Autodesk Fusion 360 part; units mm, degrees
(part 6 of 6)
sketch "plate_coriander" plane through (0, 10, 0) normal (0, 1, 0) x (-1, 0, 0)
  circle A0 centre (-0.9751, 69.925) radius 1.25
  circle A1 centre (-222.8626, 69.925) radius 1.25
  circle A2 centre (-0.9749, -12.775) radius 1.25
  circle A3 centre (-222.8624, -12.775) radius 1.25
  arc A4 (-213.146, 67.7514) -> (-210.5474, 66.675) centre (-210.5474, 70.35) ccw
  line L0 (-213.146, 67.7514) -> (-217.2861, 71.8915)
  arc A5 (-217.2861, 71.8915) -> (-219.1776, 72.675) centre (-219.1776, 70) ccw
  line L1 (-219.1776, 72.675) -> (-226.5474, 72.675)
  arc A6 (-226.5474, 72.675) -> (-228.4389, 71.8915) centre (-226.5474, 70) ccw
  line L2 (-228.4389, 71.8915) -> (-232.579, 67.7514)
  arc A7 (-232.579, 67.7514) -> (-233.3625, 65.8599) centre (-230.6875, 65.8599) ccw
  line L3 (-233.3625, 65.8599) -> (-233.3625, -8.7099)
  arc A8 (-233.3625, -8.7099) -> (-232.579, -10.6014) centre (-230.6875, -8.7099) ccw
  line L4 (-232.579, -10.6014) -> (-228.4389, -14.7415)
  arc A9 (-228.4389, -14.7415) -> (-226.5474, -15.525) centre (-226.5474, -12.85) ccw
  line L5 (-226.5474, -15.525) -> (-219.1776, -15.525)
  arc A10 (-219.1776, -15.525) -> (-217.2861, -14.7415) centre (-219.1776, -12.85) ccw
  line L6 (-217.2861, -14.7415) -> (-213.114, -10.5694)
  arc A11 (-213.114, -10.5694) -> (-213.1139, -10.5697) centre (-210.5375, -9.85) ccw
  arc A12 (-210.5474, -9.525) -> (-213.1139, -10.5697) centre (-210.5474, -13.2) ccw
  line L7 (-210.5474, -9.525) -> (-13.2901, -9.525)
  arc A13 (-10.6915, -10.6014) -> (-13.2901, -9.525) centre (-13.2901, -13.2) ccw
  line L8 (-10.6915, -10.6014) -> (-6.5514, -14.7415)
  arc A14 (-6.5514, -14.7415) -> (-4.6599, -15.525) centre (-4.6599, -12.85) ccw
  line L9 (-4.6599, -15.525) -> (2.7099, -15.525)
  arc A15 (2.7099, -15.525) -> (4.6014, -14.7415) centre (2.7099, -12.85) ccw
  line L10 (4.6014, -14.7415) -> (8.7415, -10.6014)
  arc A16 (8.7415, -10.6014) -> (9.525, -8.7099) centre (6.85, -8.7099) ccw
  line L11 (9.525, -8.7099) -> (9.525, 65.8599)
  arc A17 (9.525, 65.8599) -> (8.7415, 67.7514) centre (6.85, 65.8599) ccw
  line L12 (8.7415, 67.7514) -> (4.6014, 71.8915)
  arc A18 (4.6014, 71.8915) -> (2.7099, 72.675) centre (2.7099, 70) ccw
  line L13 (2.7099, 72.675) -> (-4.6599, 72.675)
  arc A19 (-4.6599, 72.675) -> (-6.5514, 71.8915) centre (-4.6599, 70) ccw
  line L14 (-6.5514, 71.8915) -> (-10.6915, 67.7514)
  arc A20 (-13.2901, 66.675) -> (-10.6915, 67.7514) centre (-13.2901, 70.35) ccw
  line L15 (-13.2901, 66.675) -> (-210.5474, 66.675)
  line L16 (-88.25, 26.05) -> (-88.25, 12.05)
  line L17 (-88.25, 12.05) -> (-102.25, 12.05)
  line L18 (-102.25, 12.05) -> (-102.25, 26.05)
  line L19 (-102.25, 26.05) -> (-88.25, 26.05)
  line L20 (-230.8375, 45.1) -> (-216.8375, 45.1)
  line L21 (-216.8375, 45.1) -> (-216.8375, 31.1)
  line L22 (-216.8375, 31.1) -> (-230.8375, 31.1)
  line L23 (-230.8375, 31.1) -> (-230.8375, 45.1)
  line L24 (-50.15, 31.1) -> (-64.15, 31.1)
  line L25 (-64.15, 31.1) -> (-64.15, 45.1)
  line L26 (-64.15, 45.1) -> (-50.15, 45.1)
  line L27 (-50.15, 45.1) -> (-50.15, 31.1)
  line L28 (-57.0063, 64.15) -> (-43.0063, 64.15)
  line L29 (-43.0063, 64.15) -> (-43.0063, 50.15)
  line L30 (-43.0063, 50.15) -> (-57.0063, 50.15)
  line L31 (-57.0063, 50.15) -> (-57.0063, 64.15)
  line L32 (-140.6375, 26.05) -> (-140.6375, 12.05)
  line L33 (-140.6375, 12.05) -> (-154.6375, 12.05)
  line L34 (-154.6375, 12.05) -> (-154.6375, 26.05)
  line L35 (-154.6375, 26.05) -> (-140.6375, 26.05)
  line L36 (-230.8375, -7) -> (-230.8375, 7)
  line L37 (-230.8375, 7) -> (-216.8375, 7)
  line L38 (-216.8375, 7) -> (-216.8375, -7)
  line L39 (-216.8375, -7) -> (-230.8375, -7)
  line L40 (-31.1, 7) -> (-31.1, -7)
  line L41 (-31.1, -7) -> (-45.1, -7)
  line L42 (-45.1, -7) -> (-45.1, 7)
  line L43 (-45.1, 7) -> (-31.1, 7)
  line L44 (-211.7875, 45.1) -> (-197.7875, 45.1)
  line L45 (-197.7875, 45.1) -> (-197.7875, 31.1)
  line L46 (-197.7875, 31.1) -> (-211.7875, 31.1)
  line L47 (-211.7875, 31.1) -> (-211.7875, 45.1)
  line L48 (-12.05, 26.05) -> (-12.05, 12.05)
  line L49 (-12.05, 12.05) -> (-26.05, 12.05)
  line L50 (-26.05, 12.05) -> (-26.05, 26.05)
  line L51 (-26.05, 26.05) -> (-12.05, 26.05)
  line L52 (-26.05, -7) -> (-26.05, 7)
  line L53 (-26.05, 7) -> (-12.05, 7)
  line L54 (-12.05, 7) -> (-12.05, -7)
  line L55 (-12.05, -7) -> (-26.05, -7)
  line L56 (-128.4437, 31.1) -> (-128.4437, 45.1)
  line L57 (-128.4437, 45.1) -> (-114.4438, 45.1)
  line L58 (-114.4438, 45.1) -> (-114.4438, 31.1)
  line L59 (-114.4438, 31.1) -> (-128.4437, 31.1)
  line L60 (-140.6375, 7) -> (-140.6375, -7)
  line L61 (-140.6375, -7) -> (-154.6375, -7)
  line L62 (-154.6375, -7) -> (-154.6375, 7)
  line L63 (-154.6375, 7) -> (-140.6375, 7)
  line L64 (-192.7375, 12.05) -> (-192.7375, 26.05)
  line L65 (-192.7375, 26.05) -> (-178.7375, 26.05)
  line L66 (-178.7375, 26.05) -> (-178.7375, 12.05)
  line L67 (-178.7375, 12.05) -> (-192.7375, 12.05)
  line L68 (-173.6875, 45.1) -> (-159.6875, 45.1)
  line L69 (-159.6875, 45.1) -> (-159.6875, 31.1)
  line L70 (-159.6875, 31.1) -> (-173.6875, 31.1)
  line L71 (-173.6875, 31.1) -> (-173.6875, 45.1)
  line L72 (-159.6875, -7) -> (-173.6875, -7)
  line L73 (-173.6875, -7) -> (-173.6875, 7)
  line L74 (-173.6875, 7) -> (-159.6875, 7)
  line L75 (-159.6875, 7) -> (-159.6875, -7)
  line L76 (-50.15, 26.05) -> (-50.15, 12.05)
  line L77 (-50.15, 12.05) -> (-64.15, 12.05)
  line L78 (-64.15, 12.05) -> (-64.15, 26.05)
  line L79 (-64.15, 26.05) -> (-50.15, 26.05)
  line L80 (-19.1938, 50.15) -> (-33.1938, 50.15)
  line L81 (-33.1938, 50.15) -> (-33.1938, 64.15)
  line L82 (-33.1938, 64.15) -> (-19.1938, 64.15)
  line L83 (-19.1938, 64.15) -> (-19.1938, 50.15)
  line L84 (-192.7375, 7) -> (-178.7375, 7)
  line L85 (-178.7375, 7) -> (-178.7375, -7)
  line L86 (-178.7375, -7) -> (-192.7375, -7)
  line L87 (-192.7375, -7) -> (-192.7375, 7)
  line L88 (-69.2, 7) -> (-69.2, -7)
  line L89 (-69.2, -7) -> (-83.2, -7)
  line L90 (-83.2, -7) -> (-83.2, 7)
  line L91 (-83.2, 7) -> (-69.2, 7)
  line L92 (-133.4938, 64.15) -> (-133.4938, 50.15)
  line L93 (-133.4938, 50.15) -> (-148.9318, 50.15)
  line L94 (-148.9317, 50.15) -> (-148.9317, 49.15)
  line L95 (-148.9317, 49.15) -> (-155.9317, 49.15)
  line L96 (-155.9317, 49.15) -> (-155.9317, 64.15)
  line L97 (-155.9317, 64.15) -> (-133.4938, 64.15)
  line L98 (-88.25, -7) -> (-102.25, -7)
  line L99 (-102.25, -7) -> (-102.25, 7)
  line L100 (-102.25, 7) -> (-88.25, 7)
  line L101 (-88.25, 7) -> (-88.25, -7)
  line L102 (-211.7875, 7) -> (-197.7875, 7)
  line L103 (-197.7875, 7) -> (-197.7875, -7)
  line L104 (-197.7875, -7) -> (-211.7875, -7)
  line L105 (-211.7875, -7) -> (-211.7875, 7)
  line L106 (-173.6875, 26.05) -> (-159.6875, 26.05)
  line L107 (-159.6875, 26.05) -> (-159.6875, 12.05)
  line L108 (-159.6875, 12.05) -> (-173.6875, 12.05)
  line L109 (-173.6875, 12.05) -> (-173.6875, 26.05)
  line L110 (-50.15, -7) -> (-64.15, -7)
  line L111 (-64.15, -7) -> (-64.15, 7)
  line L112 (-64.15, 7) -> (-50.15, 7)
  line L113 (-50.15, 7) -> (-50.15, -7)
  line L114 (-216.8375, 26.05) -> (-216.8375, 12.05)
  line L115 (-216.8375, 12.05) -> (-230.8375, 12.05)
  line L116 (-230.8375, 12.05) -> (-230.8375, 26.05)
  line L117 (-230.8375, 26.05) -> (-216.8375, 26.05)
  line L118 (-128.4437, 26.05) -> (-114.4438, 26.05)
  line L119 (-114.4438, 26.05) -> (-114.4438, 12.05)
  line L120 (-114.4438, 12.05) -> (-128.4437, 12.05)
  line L121 (-128.4437, 12.05) -> (-128.4437, 26.05)
  line L122 (-154.6375, 45.1) -> (-140.6375, 45.1)
  line L123 (-140.6375, 45.1) -> (-140.6375, 31.1)
  line L124 (-140.6375, 31.1) -> (-154.6375, 31.1)
  line L125 (-154.6375, 31.1) -> (-154.6375, 45.1)
  line L126 (-69.2, 12.05) -> (-83.2, 12.05)
  line L127 (-83.2, 12.05) -> (-83.2, 26.05)
  line L128 (-83.2, 26.05) -> (-69.2, 26.05)
  line L129 (-69.2, 26.05) -> (-69.2, 12.05)
  line L130 (-178.7375, 31.1) -> (-192.7375, 31.1)
  line L131 (-192.7375, 31.1) -> (-192.7375, 45.1)
  line L132 (-192.7375, 45.1) -> (-178.7375, 45.1)
  line L133 (-178.7375, 45.1) -> (-178.7375, 31.1)
  line L134 (7, -7) -> (-7, -7)
  line L135 (-7, -7) -> (-7, 7)
  line L136 (-7, 7) -> (7, 7)
  line L137 (7, 7) -> (7, -7)
  line L138 (-45.1, 26.05) -> (-31.1, 26.05)
  line L139 (-31.1, 26.05) -> (-31.1, 12.05)
  line L140 (-31.1, 12.05) -> (-45.1, 12.05)
  line L141 (-45.1, 12.05) -> (-45.1, 26.05)
  line L142 (-74.9438, 50.15) -> (-77.4625, 50.15)
  line L143 (-77.4625, 50.15) -> (-77.4625, 49.15)
  line L144 (-77.4625, 49.15) -> (-84.4625, 49.15)
  line L145 (-84.4625, 49.15) -> (-84.4625, 50.15)
  line L146 (-84.4625, 50.15) -> (-84.5745, 50.15)
  line L147 (-84.5745, 50.15) -> (-84.5745, 49.15)
  line L148 (-84.5745, 49.15) -> (-91.5745, 49.15)
  line L149 (-91.5745, 49.15) -> (-91.5745, 50.15)
  line L150 (-91.5745, 50.15) -> (-106.0375, 50.15)
  line L151 (-106.0375, 50.15) -> (-106.0375, 49.15)
  line L152 (-106.0375, 49.15) -> (-115.4505, 49.15)
  line L153 (-115.4505, 49.15) -> (-115.4505, 50.15)
  line L154 (-115.4505, 50.15) -> (-125.0558, 50.15)
  line L155 (-125.0557, 50.15) -> (-125.0557, 49.15)
  line L156 (-125.0557, 49.15) -> (-132.0875, 49.15)
  line L157 (-132.0875, 49.15) -> (-132.0875, 64.15)
  line L158 (-132.0875, 64.15) -> (-64.4375, 64.15)
  line L159 (-64.4375, 64.15) -> (-64.4375, 50.15)
  line L160 (-64.4375, 50.15) -> (-67.9375, 50.15)
  line L161 (-67.9375, 50.15) -> (-67.9375, 49.15)
  line L162 (-67.9375, 49.15) -> (-74.9438, 49.15)
  line L163 (-74.9438, 49.15) -> (-74.9438, 50.15)
  line L164 (-163.1875, 64.15) -> (-163.1875, 49.15)
  line L165 (-163.1875, 49.15) -> (-179.7125, 49.15)
  line L166 (-179.7125, 49.15) -> (-179.7125, 50.15)
  line L167 (-179.7125, 50.15) -> (-230.8375, 50.15)
  line L168 (-230.8375, 50.15) -> (-230.8375, 64.15)
  line L169 (-230.8375, 64.15) -> (-163.1875, 64.15)
  line L170 (-31.1, 45.1) -> (-31.1, 31.1)
  line L171 (-31.1, 31.1) -> (-45.1, 31.1)
  line L172 (-45.1, 31.1) -> (-45.1, 45.1)
  line L173 (-45.1, 45.1) -> (-31.1, 45.1)
  line L174 (-9.3813, 50.15) -> (-9.3813, 64.15)
  line L175 (-9.3813, 64.15) -> (4.6187, 64.15)
  line L176 (4.6187, 64.15) -> (4.6187, 50.15)
  line L177 (4.6187, 50.15) -> (-9.3813, 50.15)
  line L178 (-69.2, 31.1) -> (-83.2, 31.1)
  line L179 (-83.2, 31.1) -> (-83.2, 45.1)
  line L180 (-83.2, 45.1) -> (-69.2, 45.1)
  line L181 (-69.2, 45.1) -> (-69.2, 31.1)
  line L182 (-114.4438, -7) -> (-128.4437, -7)
  line L183 (-128.4437, -7) -> (-128.4437, 7)
  line L184 (-128.4437, 7) -> (-114.4438, 7)
  line L185 (-114.4438, 7) -> (-114.4438, -7)
  line L186 (7, 31.1) -> (-7, 31.1)
  line L187 (-7, 31.1) -> (-7, 45.1)
  line L188 (-7, 45.1) -> (7, 45.1)
  line L189 (7, 45.1) -> (7, 31.1)
  line L190 (-7, 26.05) -> (7, 26.05)
  line L191 (7, 26.05) -> (7, 12.05)
  line L192 (7, 12.05) -> (-7, 12.05)
  line L193 (-7, 12.05) -> (-7, 26.05)
  line L194 (-88.25, 45.1) -> (-88.25, 31.1)
  line L195 (-88.25, 31.1) -> (-102.25, 31.1)
  line L196 (-102.25, 31.1) -> (-102.25, 45.1)
  line L197 (-102.25, 45.1) -> (-88.25, 45.1)
  line L198 (-26.05, 31.1) -> (-26.05, 45.1)
  line L199 (-26.05, 45.1) -> (-12.05, 45.1)
  line L200 (-12.05, 45.1) -> (-12.05, 31.1)
  line L201 (-12.05, 31.1) -> (-26.05, 31.1)
  line L202 (-211.7875, 26.05) -> (-197.7875, 26.05)
  line L203 (-197.7875, 26.05) -> (-197.7875, 12.05)
  line L204 (-197.7875, 12.05) -> (-211.7875, 12.05)
  line L205 (-211.7875, 12.05) -> (-211.7875, 26.05)
sketch "plate_hull" plane through (0, 10, 0) normal (0, 1, 0) x (-1, 0, 0)
  arc A0 (13.2825, 65.2262) -> (13.4924, 66.1114) centre (13.1854, 65.7167) ccw
  arc A1 (13.4924, 66.1114) -> (11.85, 66.675) centre (11.85, 64) ccw
  line L0 (11.85, 66.675) -> (-235.6875, 66.675)
  arc A2 (-235.6875, 66.675) -> (-237.3299, 66.1114) centre (-235.6875, 64) ccw
  arc A3 (-237.3299, 66.1114) -> (-237.12, 65.2262) centre (-237.0229, 65.7167) ccw
  arc A4 (-237.12, 62.7738) -> (-237.12, 65.2262) centre (-237.3625, 64) ccw
  arc A5 (-237.12, 62.7738) -> (-237.3299, 61.8886) centre (-237.0229, 62.2833) ccw
  arc A6 (-237.3299, 61.8886) -> (-235.6875, 61.325) centre (-235.6875, 64) ccw
  line L1 (-235.6875, 61.325) -> (-234.8625, 61.325)
  arc A7 (-233.3625, 59.825) -> (-234.8625, 61.325) centre (-234.8625, 59.825) ccw
  line L2 (-233.3625, 59.825) -> (-233.3625, -2.675)
  arc A8 (-234.8625, -4.175) -> (-233.3625, -2.675) centre (-234.8625, -2.675) ccw
  line L3 (-234.8625, -4.175) -> (-235.6875, -4.175)
  arc A9 (-235.6875, -4.175) -> (-237.3299, -4.7386) centre (-235.6875, -6.85) ccw
  arc A10 (-237.3299, -4.7386) -> (-237.12, -5.6238) centre (-237.0229, -5.1333) ccw
  arc A11 (-237.12, -8.0762) -> (-237.12, -5.6238) centre (-237.3625, -6.85) ccw
  arc A12 (-237.12, -8.0762) -> (-237.3299, -8.9614) centre (-237.0229, -8.5667) ccw
  arc A13 (-237.3299, -8.9614) -> (-235.6875, -9.525) centre (-235.6875, -6.85) ccw
  line L4 (-235.6875, -9.525) -> (11.85, -9.525)
  arc A14 (11.85, -9.525) -> (13.4924, -8.9614) centre (11.85, -6.85) ccw
  arc A15 (13.4924, -8.9614) -> (13.2825, -8.0762) centre (13.1854, -8.5667) ccw
  arc A16 (13.2825, -5.6238) -> (13.2825, -8.0762) centre (13.525, -6.85) ccw
  arc A17 (13.2825, -5.6238) -> (13.4924, -4.7386) centre (13.1854, -5.1333) ccw
  arc A18 (13.4924, -4.7386) -> (11.85, -4.175) centre (11.85, -6.85) ccw
  line L5 (11.85, -4.175) -> (11.025, -4.175)
  arc A19 (9.525, -2.675) -> (11.025, -4.175) centre (11.025, -2.675) ccw
  line L6 (9.525, -2.675) -> (9.525, 59.825)
  arc A20 (11.025, 61.325) -> (9.525, 59.825) centre (11.025, 59.825) ccw
  line L7 (11.025, 61.325) -> (11.85, 61.325)
  arc A21 (11.85, 61.325) -> (13.4924, 61.8886) centre (11.85, 64) ccw
  arc A22 (13.4924, 61.8886) -> (13.2825, 62.7738) centre (13.1854, 62.2833) ccw
  arc A23 (13.2825, 65.2262) -> (13.2825, 62.7738) centre (13.525, 64) ccw
  line L8 (-88.25, 26.05) -> (-88.25, 12.05)
  line L9 (-88.25, 12.05) -> (-102.25, 12.05)
  line L10 (-102.25, 12.05) -> (-102.25, 26.05)
  line L11 (-102.25, 26.05) -> (-88.25, 26.05)
  line L12 (-230.8375, 45.1) -> (-216.8375, 45.1)
  line L13 (-216.8375, 45.1) -> (-216.8375, 31.1)
  line L14 (-216.8375, 31.1) -> (-230.8375, 31.1)
  line L15 (-230.8375, 31.1) -> (-230.8375, 45.1)
  line L16 (-50.15, 31.1) -> (-64.15, 31.1)
  line L17 (-64.15, 31.1) -> (-64.15, 45.1)
  line L18 (-64.15, 45.1) -> (-50.15, 45.1)
  line L19 (-50.15, 45.1) -> (-50.15, 31.1)
  line L20 (-57.0063, 64.15) -> (-43.0063, 64.15)
  line L21 (-43.0063, 64.15) -> (-43.0063, 50.15)
  line L22 (-43.0063, 50.15) -> (-57.0063, 50.15)
  line L23 (-57.0063, 50.15) -> (-57.0063, 64.15)
  line L24 (-140.6375, 26.05) -> (-140.6375, 12.05)
  line L25 (-140.6375, 12.05) -> (-154.6375, 12.05)
  line L26 (-154.6375, 12.05) -> (-154.6375, 26.05)
  line L27 (-154.6375, 26.05) -> (-140.6375, 26.05)
  line L28 (-230.8375, -7) -> (-230.8375, 7)
  line L29 (-230.8375, 7) -> (-216.8375, 7)
  line L30 (-216.8375, 7) -> (-216.8375, -7)
  line L31 (-216.8375, -7) -> (-230.8375, -7)
  line L32 (-31.1, 7) -> (-31.1, -7)
  line L33 (-31.1, -7) -> (-45.1, -7)
  line L34 (-45.1, -7) -> (-45.1, 7)
  line L35 (-45.1, 7) -> (-31.1, 7)
  line L36 (-211.7875, 45.1) -> (-197.7875, 45.1)
  line L37 (-197.7875, 45.1) -> (-197.7875, 31.1)
  line L38 (-197.7875, 31.1) -> (-211.7875, 31.1)
  line L39 (-211.7875, 31.1) -> (-211.7875, 45.1)
  line L40 (-12.05, 26.05) -> (-12.05, 12.05)
  line L41 (-12.05, 12.05) -> (-26.05, 12.05)
  line L42 (-26.05, 12.05) -> (-26.05, 26.05)
  line L43 (-26.05, 26.05) -> (-12.05, 26.05)
  line L44 (-26.05, -7) -> (-26.05, 7)
  line L45 (-26.05, 7) -> (-12.05, 7)
  line L46 (-12.05, 7) -> (-12.05, -7)
  line L47 (-12.05, -7) -> (-26.05, -7)
  line L48 (-128.4437, 31.1) -> (-128.4437, 45.1)
  line L49 (-128.4437, 45.1) -> (-114.4438, 45.1)
  line L50 (-114.4438, 45.1) -> (-114.4438, 31.1)
  line L51 (-114.4438, 31.1) -> (-128.4437, 31.1)
  line L52 (-140.6375, 7) -> (-140.6375, -7)
  line L53 (-140.6375, -7) -> (-154.6375, -7)
  line L54 (-154.6375, -7) -> (-154.6375, 7)
  line L55 (-154.6375, 7) -> (-140.6375, 7)
  line L56 (-192.7375, 12.05) -> (-192.7375, 26.05)
  line L57 (-192.7375, 26.05) -> (-178.7375, 26.05)
  line L58 (-178.7375, 26.05) -> (-178.7375, 12.05)
  line L59 (-178.7375, 12.05) -> (-192.7375, 12.05)
  line L60 (-173.6875, 45.1) -> (-159.6875, 45.1)
  line L61 (-159.6875, 45.1) -> (-159.6875, 31.1)
  line L62 (-159.6875, 31.1) -> (-173.6875, 31.1)
  line L63 (-173.6875, 31.1) -> (-173.6875, 45.1)
  line L64 (-159.6875, -7) -> (-173.6875, -7)
  line L65 (-173.6875, -7) -> (-173.6875, 7)
  line L66 (-173.6875, 7) -> (-159.6875, 7)
  line L67 (-159.6875, 7) -> (-159.6875, -7)
  line L68 (-50.15, 26.05) -> (-50.15, 12.05)
  line L69 (-50.15, 12.05) -> (-64.15, 12.05)
  line L70 (-64.15, 12.05) -> (-64.15, 26.05)
  line L71 (-64.15, 26.05) -> (-50.15, 26.05)
  line L72 (-19.1938, 50.15) -> (-33.1938, 50.15)
  line L73 (-33.1938, 50.15) -> (-33.1938, 64.15)
  line L74 (-33.1938, 64.15) -> (-19.1938, 64.15)
  line L75 (-19.1938, 64.15) -> (-19.1938, 50.15)
  line L76 (-192.7375, 7) -> (-178.7375, 7)
  line L77 (-178.7375, 7) -> (-178.7375, -7)
  line L78 (-178.7375, -7) -> (-192.7375, -7)
  line L79 (-192.7375, -7) -> (-192.7375, 7)
  line L80 (-69.2, 7) -> (-69.2, -7)
  line L81 (-69.2, -7) -> (-83.2, -7)
  line L82 (-83.2, -7) -> (-83.2, 7)
  line L83 (-83.2, 7) -> (-69.2, 7)
  line L84 (-133.4938, 64.15) -> (-133.4938, 50.15)
  line L85 (-133.4938, 50.15) -> (-148.9318, 50.15)
  line L86 (-148.9317, 50.15) -> (-148.9317, 49.15)
  line L87 (-148.9317, 49.15) -> (-155.9317, 49.15)
  line L88 (-155.9317, 49.15) -> (-155.9317, 64.15)
  line L89 (-155.9317, 64.15) -> (-133.4938, 64.15)
  line L90 (-88.25, -7) -> (-102.25, -7)
  line L91 (-102.25, -7) -> (-102.25, 7)
  line L92 (-102.25, 7) -> (-88.25, 7)
  line L93 (-88.25, 7) -> (-88.25, -7)
  line L94 (-211.7875, 7) -> (-197.7875, 7)
  line L95 (-197.7875, 7) -> (-197.7875, -7)
  line L96 (-197.7875, -7) -> (-211.7875, -7)
  line L97 (-211.7875, -7) -> (-211.7875, 7)
  line L98 (-173.6875, 26.05) -> (-159.6875, 26.05)
  line L99 (-159.6875, 26.05) -> (-159.6875, 12.05)
  line L100 (-159.6875, 12.05) -> (-173.6875, 12.05)
  line L101 (-173.6875, 12.05) -> (-173.6875, 26.05)
  line L102 (-50.15, -7) -> (-64.15, -7)
  line L103 (-64.15, -7) -> (-64.15, 7)
  line L104 (-64.15, 7) -> (-50.15, 7)
  line L105 (-50.15, 7) -> (-50.15, -7)
  line L106 (-216.8375, 26.05) -> (-216.8375, 12.05)
  line L107 (-216.8375, 12.05) -> (-230.8375, 12.05)
  line L108 (-230.8375, 12.05) -> (-230.8375, 26.05)
  line L109 (-230.8375, 26.05) -> (-216.8375, 26.05)
  line L110 (-128.4437, 26.05) -> (-114.4438, 26.05)
  line L111 (-114.4438, 26.05) -> (-114.4438, 12.05)
  line L112 (-114.4438, 12.05) -> (-128.4437, 12.05)
  line L113 (-128.4437, 12.05) -> (-128.4437, 26.05)
  line L114 (-154.6375, 45.1) -> (-140.6375, 45.1)
  line L115 (-140.6375, 45.1) -> (-140.6375, 31.1)
  line L116 (-140.6375, 31.1) -> (-154.6375, 31.1)
  line L117 (-154.6375, 31.1) -> (-154.6375, 45.1)
  line L118 (-69.2, 12.05) -> (-83.2, 12.05)
  line L119 (-83.2, 12.05) -> (-83.2, 26.05)
  line L120 (-83.2, 26.05) -> (-69.2, 26.05)
  line L121 (-69.2, 26.05) -> (-69.2, 12.05)
  line L122 (-178.7375, 31.1) -> (-192.7375, 31.1)
  line L123 (-192.7375, 31.1) -> (-192.7375, 45.1)
  line L124 (-192.7375, 45.1) -> (-178.7375, 45.1)
  line L125 (-178.7375, 45.1) -> (-178.7375, 31.1)
  line L126 (7, -7) -> (-7, -7)
  line L127 (-7, -7) -> (-7, 7)
  line L128 (-7, 7) -> (7, 7)
  line L129 (7, 7) -> (7, -7)
  line L130 (-45.1, 26.05) -> (-31.1, 26.05)
  line L131 (-31.1, 26.05) -> (-31.1, 12.05)
  line L132 (-31.1, 12.05) -> (-45.1, 12.05)
  line L133 (-45.1, 12.05) -> (-45.1, 26.05)
  line L134 (-74.9438, 50.15) -> (-77.4625, 50.15)
  line L135 (-77.4625, 50.15) -> (-77.4625, 49.15)
  line L136 (-77.4625, 49.15) -> (-84.4625, 49.15)
  line L137 (-84.4625, 49.15) -> (-84.4625, 50.15)
  line L138 (-84.4625, 50.15) -> (-84.5745, 50.15)
  line L139 (-84.5745, 50.15) -> (-84.5745, 49.15)
  line L140 (-84.5745, 49.15) -> (-91.5745, 49.15)
  line L141 (-91.5745, 49.15) -> (-91.5745, 50.15)
  line L142 (-91.5745, 50.15) -> (-106.0375, 50.15)
  line L143 (-106.0375, 50.15) -> (-106.0375, 49.15)
  line L144 (-106.0375, 49.15) -> (-115.4505, 49.15)
  line L145 (-115.4505, 49.15) -> (-115.4505, 50.15)
  line L146 (-115.4505, 50.15) -> (-125.0558, 50.15)
  line L147 (-125.0557, 50.15) -> (-125.0557, 49.15)
  line L148 (-125.0557, 49.15) -> (-132.0875, 49.15)
  line L149 (-132.0875, 49.15) -> (-132.0875, 64.15)
  line L150 (-132.0875, 64.15) -> (-64.4375, 64.15)
  line L151 (-64.4375, 64.15) -> (-64.4375, 50.15)
  line L152 (-64.4375, 50.15) -> (-67.9375, 50.15)
  line L153 (-67.9375, 50.15) -> (-67.9375, 49.15)
  line L154 (-67.9375, 49.15) -> (-74.9438, 49.15)
  line L155 (-74.9438, 49.15) -> (-74.9438, 50.15)
  line L156 (-163.1875, 64.15) -> (-163.1875, 49.15)
  line L157 (-163.1875, 49.15) -> (-179.7125, 49.15)
  line L158 (-179.7125, 49.15) -> (-179.7125, 50.15)
  line L159 (-179.7125, 50.15) -> (-230.8375, 50.15)
  line L160 (-230.8375, 50.15) -> (-230.8375, 64.15)
  line L161 (-230.8375, 64.15) -> (-163.1875, 64.15)
  line L162 (-31.1, 45.1) -> (-31.1, 31.1)
  line L163 (-31.1, 31.1) -> (-45.1, 31.1)
  line L164 (-45.1, 31.1) -> (-45.1, 45.1)
  line L165 (-45.1, 45.1) -> (-31.1, 45.1)
  line L166 (-9.3813, 50.15) -> (-9.3813, 64.15)
  line L167 (-9.3813, 64.15) -> (4.6187, 64.15)
  line L168 (4.6187, 64.15) -> (4.6187, 50.15)
  line L169 (4.6187, 50.15) -> (-9.3813, 50.15)
  line L170 (-69.2, 31.1) -> (-83.2, 31.1)
  line L171 (-83.2, 31.1) -> (-83.2, 45.1)
  line L172 (-83.2, 45.1) -> (-69.2, 45.1)
  line L173 (-69.2, 45.1) -> (-69.2, 31.1)
  line L174 (-114.4438, -7) -> (-128.4437, -7)
  line L175 (-128.4437, -7) -> (-128.4437, 7)
  line L176 (-128.4437, 7) -> (-114.4438, 7)
  line L177 (-114.4438, 7) -> (-114.4438, -7)
  line L178 (7, 31.1) -> (-7, 31.1)
  line L179 (-7, 31.1) -> (-7, 45.1)
  line L180 (-7, 45.1) -> (7, 45.1)
  line L181 (7, 45.1) -> (7, 31.1)
  line L182 (-7, 26.05) -> (7, 26.05)
  line L183 (7, 26.05) -> (7, 12.05)
  line L184 (7, 12.05) -> (-7, 12.05)
  line L185 (-7, 12.05) -> (-7, 26.05)
  line L186 (-88.25, 45.1) -> (-88.25, 31.1)
  line L187 (-88.25, 31.1) -> (-102.25, 31.1)
  line L188 (-102.25, 31.1) -> (-102.25, 45.1)
  line L189 (-102.25, 45.1) -> (-88.25, 45.1)
  line L190 (-26.05, 31.1) -> (-26.05, 45.1)
  line L191 (-26.05, 45.1) -> (-12.05, 45.1)
  line L192 (-12.05, 45.1) -> (-12.05, 31.1)
  line L193 (-12.05, 31.1) -> (-26.05, 31.1)
  line L194 (-211.7875, 26.05) -> (-197.7875, 26.05)
  line L195 (-197.7875, 26.05) -> (-197.7875, 12.05)
  line L196 (-197.7875, 12.05) -> (-211.7875, 12.05)
  line L197 (-211.7875, 12.05) -> (-211.7875, 26.05)
sketch "plate_tray" plane through (0, 10, 0) normal (0, 1, 0) x (-1, 0, 0)
  arc A0 (-20.7867, 7) -> (-20.7844, 12.05) centre (-21.875, 9.5255) ccw
  arc A1 (-127.5983, 26.05) -> (-127.3626, 31.1) centre (-128.5623, 28.6255) ccw
  arc A2 (-96.9867, 7) -> (-96.9844, 12.05) centre (-98.075, 9.5255) ccw
  line L0 (9.775, -6.5245) -> (9.775, 63.6754)
  arc A3 (9.775, 63.6754) -> (6.775, 66.6754) centre (6.775, 63.6754) ccw
  line L1 (6.775, 66.6754) -> (-230.6123, 66.6754)
  arc A4 (-230.6123, 66.6754) -> (-233.6123, 63.6754) centre (-230.6123, 63.6754) ccw
  line L2 (-233.6123, 63.6754) -> (-233.6123, -6.5245)
  arc A5 (-233.6123, -6.5245) -> (-230.6123, -9.5245) centre (-230.6123, -6.5245) ccw
  line L3 (-230.6123, -9.5245) -> (6.775, -9.5245)
  arc A6 (6.775, -9.5245) -> (9.775, -6.5245) centre (6.775, -6.5245) ccw
  line L4 (-128.4437, 31.3729) -> (-128.4437, 45.1)
  line L5 (-128.4437, 45.1) -> (-114.4438, 45.1)
  line L6 (-114.4438, 45.1) -> (-114.4438, 31.1)
  line L7 (-114.4438, 31.1) -> (-127.3626, 31.1)
  line L8 (-127.5983, 26.05) -> (-114.4438, 26.05)
  line L9 (-114.4438, 26.05) -> (-114.4438, 12.05)
  line L10 (-114.4438, 12.05) -> (-128.4437, 12.05)
  line L11 (-128.4437, 12.05) -> (-128.4437, 25.8781)
  arc A7 (-128.4437, 31.3729) -> (-128.4437, 25.8781) centre (-128.5623, 28.6255) ccw
  line L12 (-198.3716, 7) -> (-197.7875, 7)
  line L13 (-197.7875, 7) -> (-197.7875, -7)
  line L14 (-197.7875, -7) -> (-211.7875, -7)
  line L15 (-211.7875, -7) -> (-211.7875, 7)
  line L16 (-211.7875, 7) -> (-203.853, 7)
  arc A8 (-198.3716, 7) -> (-203.853, 7) centre (-201.1123, 7.2255) ccw
  line L17 (-17.7015, 45.1) -> (-12.05, 45.1)
  line L18 (-12.05, 45.1) -> (-12.05, 31.1)
  line L19 (-12.05, 31.1) -> (-26.05, 31.1)
  line L20 (-26.05, 31.1) -> (-26.05, 45.1)
  line L21 (-26.05, 45.1) -> (-22.9485, 45.1)
  arc A9 (-17.7015, 45.1) -> (-22.9485, 45.1) centre (-20.325, 44.2754) ccw
  line L22 (-211.7875, 26.05) -> (-197.7875, 26.05)
  line L23 (-197.7875, 26.05) -> (-197.7875, 12.05)
  line L24 (-197.7875, 12.05) -> (-211.7875, 12.05)
  line L25 (-211.7875, 12.05) -> (-211.7875, 26.05)
  line L26 (-88.25, 45.1) -> (-88.25, 31.1)
  line L27 (-88.25, 31.1) -> (-102.25, 31.1)
  line L28 (-102.25, 31.1) -> (-102.25, 45.1)
  line L29 (-102.25, 45.1) -> (-88.25, 45.1)
  line L30 (-7, 26.05) -> (7, 26.05)
  line L31 (7, 26.05) -> (7, 12.05)
  line L32 (7, 12.05) -> (-7, 12.05)
  line L33 (-7, 12.05) -> (-7, 26.05)
  line L34 (7, 31.1) -> (-7, 31.1)
  line L35 (-7, 31.1) -> (-7, 45.1)
  line L36 (-7, 45.1) -> (7, 45.1)
  line L37 (7, 45.1) -> (7, 31.1)
  line L38 (-114.4438, -7) -> (-128.4437, -7)
  line L39 (-128.4437, -7) -> (-128.4437, 7)
  line L40 (-128.4437, 7) -> (-114.4438, 7)
  line L41 (-114.4438, 7) -> (-114.4438, -7)
  line L42 (-69.2, 31.1) -> (-83.2, 31.1)
  line L43 (-83.2, 31.1) -> (-83.2, 45.1)
  line L44 (-83.2, 45.1) -> (-69.2, 45.1)
  line L45 (-69.2, 45.1) -> (-69.2, 31.1)
  line L46 (-9.3813, 50.15) -> (-9.3813, 64.15)
  line L47 (-9.3813, 64.15) -> (4.6187, 64.15)
  line L48 (4.6187, 64.15) -> (4.6187, 50.15)
  line L49 (4.6187, 50.15) -> (-9.3813, 50.15)
  line L50 (-31.1, 45.1) -> (-31.1, 31.1)
  line L51 (-31.1, 31.1) -> (-45.1, 31.1)
  line L52 (-45.1, 31.1) -> (-45.1, 45.1)
  line L53 (-45.1, 45.1) -> (-31.1, 45.1)
  line L54 (-163.1875, 64.15) -> (-163.1875, 49.15)
  line L55 (-163.1875, 49.15) -> (-179.7125, 49.15)
  line L56 (-179.7125, 49.15) -> (-179.7125, 50.15)
  line L57 (-179.7125, 50.15) -> (-230.8375, 50.15)
  line L58 (-230.8375, 50.15) -> (-230.8375, 64.15)
  line L59 (-230.8375, 64.15) -> (-163.1875, 64.15)
  line L60 (-74.9438, 50.15) -> (-77.4625, 50.15)
  line L61 (-77.4625, 50.15) -> (-77.4625, 49.15)
  line L62 (-77.4625, 49.15) -> (-84.4625, 49.15)
  line L63 (-84.4625, 49.15) -> (-84.4625, 50.15)
  line L64 (-84.4625, 50.15) -> (-84.5745, 50.15)
  line L65 (-84.5745, 50.15) -> (-84.5745, 49.15)
  line L66 (-84.5745, 49.15) -> (-91.5745, 49.15)
  line L67 (-91.5745, 49.15) -> (-91.5745, 50.15)
  line L68 (-91.5745, 50.15) -> (-106.0375, 50.15)
  line L69 (-106.0375, 50.15) -> (-106.0375, 49.15)
  line L70 (-106.0375, 49.15) -> (-115.4505, 49.15)
  line L71 (-115.4505, 49.15) -> (-115.4505, 50.15)
  line L72 (-115.4505, 50.15) -> (-125.0558, 50.15)
  line L73 (-125.0557, 50.15) -> (-125.0557, 49.15)
  line L74 (-125.0557, 49.15) -> (-132.0875, 49.15)
  line L75 (-132.0875, 49.15) -> (-132.0875, 64.15)
  line L76 (-132.0875, 64.15) -> (-64.4375, 64.15)
  line L77 (-64.4375, 64.15) -> (-64.4375, 50.15)
  line L78 (-64.4375, 50.15) -> (-67.9375, 50.15)
  line L79 (-67.9375, 50.15) -> (-67.9375, 49.15)
  line L80 (-67.9375, 49.15) -> (-74.9438, 49.15)
  line L81 (-74.9438, 49.15) -> (-74.9438, 50.15)
  line L82 (-45.1, 26.05) -> (-31.1, 26.05)
  line L83 (-31.1, 26.05) -> (-31.1, 12.05)
  line L84 (-31.1, 12.05) -> (-45.1, 12.05)
  line L85 (-45.1, 12.05) -> (-45.1, 26.05)
  line L86 (7, -7) -> (-7, -7)
  line L87 (-7, -7) -> (-7, 7)
  line L88 (-7, 7) -> (7, 7)
  line L89 (7, 7) -> (7, -7)
  line L90 (-178.7375, 31.1) -> (-192.7375, 31.1)
  line L91 (-192.7375, 31.1) -> (-192.7375, 45.1)
  line L92 (-192.7375, 45.1) -> (-178.7375, 45.1)
  line L93 (-178.7375, 45.1) -> (-178.7375, 31.1)
  line L94 (-69.2, 12.05) -> (-83.2, 12.05)
  line L95 (-83.2, 12.05) -> (-83.2, 26.05)
  line L96 (-83.2, 26.05) -> (-69.2, 26.05)
  line L97 (-69.2, 26.05) -> (-69.2, 12.05)
  line L98 (-154.6375, 45.1) -> (-140.6375, 45.1)
  line L99 (-140.6375, 45.1) -> (-140.6375, 31.1)
  line L100 (-140.6375, 31.1) -> (-154.6375, 31.1)
  line L101 (-154.6375, 31.1) -> (-154.6375, 45.1)
  line L102 (-216.8375, 26.05) -> (-216.8375, 12.05)
  line L103 (-216.8375, 12.05) -> (-230.8375, 12.05)
  line L104 (-230.8375, 12.05) -> (-230.8375, 26.05)
  line L105 (-230.8375, 26.05) -> (-216.8375, 26.05)
  line L106 (-50.15, -7) -> (-64.15, -7)
  line L107 (-64.15, -7) -> (-64.15, 7)
  line L108 (-64.15, 7) -> (-50.15, 7)
  line L109 (-50.15, 7) -> (-50.15, -7)
  line L110 (-173.6875, 26.05) -> (-159.6875, 26.05)
  line L111 (-159.6875, 26.05) -> (-159.6875, 12.05)
  line L112 (-159.6875, 12.05) -> (-173.6875, 12.05)
  line L113 (-173.6875, 12.05) -> (-173.6875, 26.05)
  line L114 (-133.4938, 64.15) -> (-133.4938, 50.15)
  line L115 (-133.4938, 50.15) -> (-148.9318, 50.15)
  line L116 (-148.9317, 50.15) -> (-148.9317, 49.15)
  line L117 (-148.9317, 49.15) -> (-155.9317, 49.15)
  line L118 (-155.9317, 49.15) -> (-155.9317, 64.15)
  line L119 (-155.9317, 64.15) -> (-133.4938, 64.15)
  line L120 (-69.2, 7) -> (-69.2, -7)
  line L121 (-69.2, -7) -> (-83.2, -7)
  line L122 (-83.2, -7) -> (-83.2, 7)
  line L123 (-83.2, 7) -> (-69.2, 7)
  line L124 (-192.7375, 7) -> (-178.7375, 7)
  line L125 (-178.7375, 7) -> (-178.7375, -7)
  line L126 (-178.7375, -7) -> (-192.7375, -7)
  line L127 (-192.7375, -7) -> (-192.7375, 7)
  line L128 (-19.1938, 50.15) -> (-33.1938, 50.15)
  line L129 (-33.1938, 50.15) -> (-33.1938, 64.15)
  line L130 (-33.1938, 64.15) -> (-19.1938, 64.15)
  line L131 (-19.1938, 64.15) -> (-19.1938, 50.15)
  line L132 (-50.15, 26.05) -> (-50.15, 12.05)
  line L133 (-50.15, 12.05) -> (-64.15, 12.05)
  line L134 (-64.15, 12.05) -> (-64.15, 26.05)
  line L135 (-64.15, 26.05) -> (-50.15, 26.05)
  line L136 (-159.6875, -7) -> (-173.6875, -7)
  line L137 (-173.6875, -7) -> (-173.6875, 7)
  line L138 (-173.6875, 7) -> (-159.6875, 7)
  line L139 (-159.6875, 7) -> (-159.6875, -7)
  line L140 (-173.6875, 45.1) -> (-159.6875, 45.1)
  line L141 (-159.6875, 45.1) -> (-159.6875, 31.1)
  line L142 (-159.6875, 31.1) -> (-173.6875, 31.1)
  line L143 (-173.6875, 31.1) -> (-173.6875, 45.1)
  line L144 (-192.7375, 12.05) -> (-192.7375, 26.05)
  line L145 (-192.7375, 26.05) -> (-178.7375, 26.05)
  line L146 (-178.7375, 26.05) -> (-178.7375, 12.05)
  line L147 (-178.7375, 12.05) -> (-192.7375, 12.05)
  line L148 (-140.6375, 7) -> (-140.6375, -7)
  line L149 (-140.6375, -7) -> (-154.6375, -7)
  line L150 (-154.6375, -7) -> (-154.6375, 7)
  line L151 (-154.6375, 7) -> (-140.6375, 7)
  line L152 (-211.7875, 45.1) -> (-197.7875, 45.1)
  line L153 (-197.7875, 45.1) -> (-197.7875, 31.1)
  line L154 (-197.7875, 31.1) -> (-211.7875, 31.1)
  line L155 (-211.7875, 31.1) -> (-211.7875, 45.1)
  line L156 (-31.1, 7) -> (-31.1, -7)
  line L157 (-31.1, -7) -> (-45.1, -7)
  line L158 (-45.1, -7) -> (-45.1, 7)
  line L159 (-45.1, 7) -> (-31.1, 7)
  line L160 (-230.8375, -7) -> (-230.8375, 7)
  line L161 (-230.8375, 7) -> (-216.8375, 7)
  line L162 (-216.8375, 7) -> (-216.8375, -7)
  line L163 (-216.8375, -7) -> (-230.8375, -7)
  line L164 (-140.6375, 26.05) -> (-140.6375, 12.05)
  line L165 (-140.6375, 12.05) -> (-154.6375, 12.05)
  line L166 (-154.6375, 12.05) -> (-154.6375, 26.05)
  line L167 (-154.6375, 26.05) -> (-140.6375, 26.05)
  line L168 (-57.0063, 64.15) -> (-43.0063, 64.15)
  line L169 (-43.0063, 64.15) -> (-43.0063, 50.15)
  line L170 (-43.0063, 50.15) -> (-57.0063, 50.15)
  line L171 (-57.0063, 50.15) -> (-57.0063, 64.15)
  line L172 (-50.15, 31.1) -> (-64.15, 31.1)
  line L173 (-64.15, 31.1) -> (-64.15, 45.1)
  line L174 (-64.15, 45.1) -> (-50.15, 45.1)
  line L175 (-50.15, 45.1) -> (-50.15, 31.1)
  line L176 (-230.8375, 45.1) -> (-216.8375, 45.1)
  line L177 (-216.8375, 45.1) -> (-216.8375, 31.1)
  line L178 (-216.8375, 31.1) -> (-230.8375, 31.1)
  line L179 (-230.8375, 31.1) -> (-230.8375, 45.1)
  line L180 (-12.05, 12.05) -> (-20.7844, 12.05)
  line L181 (-20.7867, 7) -> (-12.05, 7)
  line L182 (-12.05, 7) -> (-12.05, -7)
  line L183 (-12.05, -7) -> (-26.05, -7)
  line L184 (-26.05, -7) -> (-26.05, 7)
  line L185 (-26.05, 7) -> (-22.9633, 7)
  arc A10 (-22.9656, 12.05) -> (-22.9633, 7) centre (-21.875, 9.5255) ccw
  line L186 (-22.9656, 12.05) -> (-26.05, 12.05)
  line L187 (-26.05, 12.05) -> (-26.05, 26.05)
  line L188 (-26.05, 26.05) -> (-12.05, 26.05)
  line L189 (-12.05, 26.05) -> (-12.05, 12.05)
  line L190 (-88.25, 12.05) -> (-96.9844, 12.05)
  line L191 (-96.9867, 7) -> (-88.25, 7)
  line L192 (-88.25, 7) -> (-88.25, -7)
  line L193 (-88.25, -7) -> (-102.25, -7)
  line L194 (-102.25, -7) -> (-102.25, 7)
  line L195 (-102.25, 7) -> (-99.1633, 7)
  arc A11 (-99.1656, 12.05) -> (-99.1633, 7) centre (-98.075, 9.5255) ccw
  line L196 (-99.1656, 12.05) -> (-102.25, 12.05)
  line L197 (-102.25, 12.05) -> (-102.25, 26.05)
  line L198 (-102.25, 26.05) -> (-88.25, 26.05)
  line L199 (-88.25, 26.05) -> (-88.25, 12.05)
hidden bodies 1 2 3 4 5 6
named bodies: "CampsiteBase", "CorianderBase", "HullBase", "TrayBase", "Campiander", "Trull"
